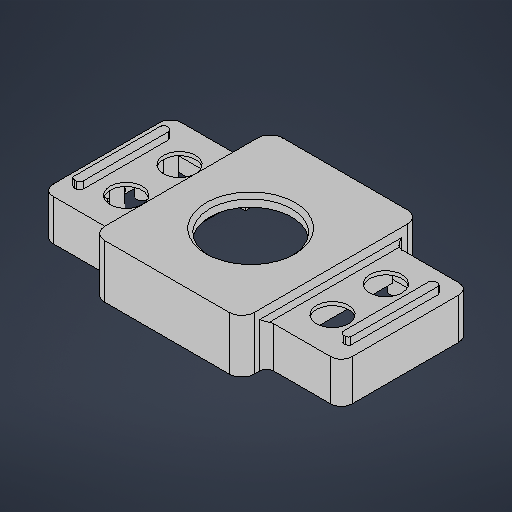
# Autodesk Inventor part: Part1
Saved by Autodesk Inventor 2026 (Build 300175000, 175)
## iProperties
Created: 2025-04-13
Part Number: Part1
Material: Generic
Document SubType Name: Modeling
Designer: ct_vi
Density: 1 g/cm^3
Appearance: Default
Author: ct_vi
Autodesk Inventor part; units mm, degrees
ref_plane "YZ Plane" through (0, 0, 0) normal (1, 0, 0) x (0, 1, 0)
ref_plane "XZ Plane" through (0, 0, 0) normal (0, 1, 0) x (-1, 0, 0)
ref_plane "XY Plane" through (0, 0, 0) normal (0, 0, 1) x (1, 0, 0)
sketch "Sketch1" plane through (0, 0, 0) normal (0, 1, 0) x (-1, 0, 0)
  circle A0 centre (0, 1.5) radius 11.5
  circle A1 centre (0, 1.5) radius 12.5
  line L0 (19.0144, -21.3297) -> (-18.8688, -21.3297) construction
  line L1 (-18.8688, -21.3297) -> (-18.8688, 21.6448) construction
  line L2 (-18.8688, 21.6448) -> (19.0144, 21.6448) construction
  line L3 (19.0144, 21.6448) -> (19.0144, -21.3297) construction
  line L4 (-2.25, -4) -> (-2.25, -8.7)
  line L5 (-2.25, -8.7) -> (2.25, -8.7)
  line L6 (2.25, -8.7) -> (2.25, -4)
  line L7 (2.25, -4) -> (-2.25, -4)
  line L8 (5.9381, 2.2148) -> (9.8353, 4.4648)
  line L9 (9.8353, 4.4648) -> (7.4853, 8.5352)
  line L10 (7.4853, 8.5352) -> (3.5881, 6.2852)
  line L11 (5.9381, 2.2148) -> (3.5881, 6.2852)
  line L12 (-3.5881, 6.2852) -> (-7.4853, 8.5352)
  line L13 (-7.4853, 8.5352) -> (-9.8353, 4.4648)
  line L14 (-9.8353, 4.4648) -> (-5.9381, 2.2148)
  line L15 (-3.5881, 6.2852) -> (-5.9381, 2.2148)
  circle A2 centre (10.199, -17.6855) radius 1.5
  circle A3 centre (-10.301, 18.0645) radius 1.5
  circle A4 centre (10.199, 18.0645) radius 1.5
  circle A5 centre (-10.301, -17.6855) radius 1.5
  line L16 (10.199, -17.6855) -> (-10.301, -17.6855)
  line L17 (-10.301, -17.6855) -> (-10.301, 18.0645)
  line L18 (-10.301, 18.0645) -> (10.199, 18.0645)
  line L19 (10.199, 18.0645) -> (10.199, -17.6855)
  line L20 (18, -22) -> (-18, -22)
  line L21 (-18, -22) -> (-18, 22)
  line L22 (-18, 22) -> (18, 22)
  line L23 (18, 22) -> (18, -22)
  line L24 (18, -22) -> (-18, 22) construction
  line L25 (-18, -22) -> (18, 22) construction
  line L26 (17.5, -25) -> (-17.5, -25)
  line L27 (-21, -21.5) -> (-21, 21.5)
  line L28 (-17.5, 25) -> (17.5, 25)
  line L29 (21, -25) -> (-21, 25) construction
  line L30 (-21, -25) -> (21, 25) construction
  arc A6 (-17.5, 25) -> (-21, 21.5) centre (-17.5, 21.5) ccw
  arc A7 (-21, -21.5) -> (-17.5, -25) centre (-17.5, -21.5) ccw
  line L31 (17.5, -23) -> (-17.5, -23)
  line L32 (-19, -21.5) -> (-19, 21.5)
  line L33 (-17.5, 23) -> (17.5, 23)
  line L34 (19, 21.5) -> (19, -21.5)
  line L35 (19, -23) -> (-19, 23) construction
  line L36 (-19, -23) -> (19, 23) construction
  arc A8 (-17.5, 23) -> (-19, 21.5) centre (-17.5, 21.5) ccw
  arc A9 (-19, -21.5) -> (-17.5, -23) centre (-17.5, -21.5) ccw
  line L37 (9.2678, 19.2405) -> (9.2678, 16.8886)
  line L38 (9.2678, -16.5095) -> (9.2678, -18.8614)
  line L39 (-9.3698, 19.2405) -> (-9.3698, 16.8886)
  line L40 (-9.3698, -16.5095) -> (-9.3698, -18.8614)
  line L41 (17.5, -24) -> (-17.5, -24)
  line L42 (-20, -21.5) -> (-20, 21.5)
  line L43 (-17.5, 24) -> (17.5, 24)
  line L44 (20, -24) -> (-20, 24) construction
  line L45 (-20, -24) -> (20, 24) construction
  arc A10 (-17.5, 24) -> (-20, 21.5) centre (-17.5, 21.5) ccw
  arc A11 (-20, -21.5) -> (-17.5, -24) centre (-17.5, -21.5) ccw
  line L46 (21, -21.5) -> (21, 21.5)
  line L47 (20, 21.5) -> (20, -21.5)
  arc A12 (17.5, -24) -> (20, -21.5) centre (17.5, -21.5) ccw
  arc A13 (17.5, -25) -> (21, -21.5) centre (17.5, -21.5) ccw
  arc A14 (17.5, -23) -> (19, -21.5) centre (17.5, -21.5) ccw
  arc A15 (21, 21.5) -> (17.5, 25) centre (17.5, 21.5) ccw
  arc A16 (20, 21.5) -> (17.5, 24) centre (17.5, 21.5) ccw
  arc A17 (19, 21.5) -> (17.5, 23) centre (17.5, 21.5) ccw
  line L48 (19, -15) -> (19, 15)
  line L49 (19, 16) -> (19, -16)
  line L50 (19, -16) -> (19, 16)
  line L51 (20, -17) -> (20, 17)
  line L52 (21, -18) -> (21, 18)
  line L53 (19, -15) -> (21.5, -15)
  line L54 (21.5, -15) -> (21.5, 16)
  line L55 (21.5, 16) -> (19, 16)
  line L56 (19, 16) -> (19, -15)
  line L57 (-19, -15) -> (-19, 15)
  line L58 (-19, -16) -> (-19, 16)
  line L59 (-21, -18) -> (-21, 19)
  line L60 (-20, -17) -> (-20, 17)
  line L61 (-20, -17) -> (-20, 17)
  line L62 (-19, -16) -> (-19, 16)
  line L63 (-19, 16) -> (-21.5, 16)
  line L64 (-21.5, 16) -> (-21.5, -16)
  line L65 (-21.5, -16) -> (-19, -16)
  line L66 (-19, -16) -> (-19, 16)
  line L67 (14, -15) -> (14, 0)
  line L68 (21, -15) -> (20, -15)
  line L69 (20, -15) -> (20, -16.5095)
  line L70 (21, -16.5095) -> (21, -15)
  line L71 (21, -15) -> (19, -15)
  line L72 (19, -15) -> (19, -16)
  line L73 (19, -16) -> (21, -16)
  line L74 (21, -16) -> (21, -15)
  line L75 (21, -16) -> (19, -16)
  line L76 (19, -16) -> (19, -17)
  line L77 (19, -17) -> (21, -17)
  line L78 (21, -17) -> (21, -16)
  line L79 (21, -17) -> (19, -17)
  line L80 (19, -17) -> (19, -18)
  line L81 (19, -18) -> (21, -18)
  line L82 (21, -18) -> (21, -17)
  line L83 (21, 16) -> (19, 16)
  line L84 (19, 16) -> (19, 18)
  line L85 (19, 18) -> (21, 18)
  line L86 (21, 18) -> (21, 16)
  line L87 (21, 18) -> (19, 18)
  line L88 (19, 18) -> (19, 19)
  line L89 (19, 19) -> (21, 19)
  line L90 (21, 19) -> (21, 18)
  line L91 (21, 18) -> (19, 18)
  line L92 (19, 18) -> (19, 17)
  line L93 (19, 17) -> (21, 17)
  line L94 (21, 17) -> (21, 18)
  line L95 (-19, 16) -> (-21, 16)
  line L96 (-21, 16) -> (-21, 17)
  line L97 (-21, 17) -> (-19, 17)
  line L98 (-19, 17) -> (-19, 16)
  line L99 (-21, 17) -> (-19, 17)
  line L100 (-19, 17) -> (-19, 18)
  line L101 (-19, 18) -> (-21, 18)
  line L102 (-21, 18) -> (-21, 17)
  line L103 (-21, 18) -> (-19, 18)
  line L104 (-19, 18) -> (-19, 19)
  line L105 (-19, 19) -> (-21, 19)
  line L106 (-21, 19) -> (-21, 18)
  line L107 (-19, -16) -> (-21, -16)
  line L108 (-21, -16) -> (-21, -17)
  line L109 (-21, -17) -> (-19, -17)
  line L110 (-19, -17) -> (-19, -16)
  line L111 (-21, -17) -> (-19, -17)
  line L112 (-19, -17) -> (-19, -18)
  line L113 (-19, -18) -> (-21, -18)
  line L114 (-21, -18) -> (-21, -17)
  line L115 (-19, -18) -> (-21, -18)
  line L116 (-21, -18) -> (-21, -19)
  line L117 (-21, -19) -> (-19, -19)
  line L118 (-19, -19) -> (-19, -18)
  point P0 (0, 0)
  point P1 (21, -22)
  point P2 (21, 22)
  point P3 (19, 24)
  point P4 (19, -24)
  point P5 (-21, -16)
  point P6 (-21, 16)
  point P7 (21, 16)
  point P8 (21, -15)
  point P9 (-20, 17)
  point P10 (20, 16)
  point P11 (20, -18)
  dimension "d33" = 4.7
  dimension "d34" = 4.5
  dimension "d36" = 4.5
  dimension "d37" = 4.7
  dimension "d38" = 3
  dimension "d46" = 3
  dimension "d47" = 3
  dimension "d48" = 3
  dimension "d211" = 1.5
  dimension "d212" = 2.5
  dimension "d216" = 3.5
  dimension "d245" = 2.5
  dimension "d246" = 3.5
  dimension "d247" = 1.5
  dimension "d248" = 3.5
  dimension "d249" = 2.5
  dimension "d250" = 1.5
  dimension "d264" = 30
  dimension "d310" = 34
  dimension "d314" = 36
  dimension "d318" = 2.5
  dimension "d366" = 2.5
  dimension "d494" = 2
  dimension "d495" = 1
  dimension "d496" = 2
  dimension "d497" = 1
  dimension "d498" = 2
  dimension "d499" = 1
  dimension "d500" = 2
  dimension "d501" = 1
  dimension "d502" = 1
  dimension "d503" = 1
  dimension "d504" = 1
  dimension "d505" = 1
  dimension "d506" = 1
  dimension "d565" = 50
  constraints: 230 end point, 45 point on line, 39 parallel, 32 point on circle, 27 perpendicular, 24 tangent, 21 horizontal, 18 centre point, 9 midpoint, 1 vertical, 2 other
  measures "d33" distance of L4.start L4.end
  measures "d34" distance of L4.end L5.end
  measures "d36" distance of L8.start L8.end
  measures "d37" distance of L8.end L9.end
  measures "d38" diameter of A2
  measures "d46" diameter of A3
  measures "d47" diameter of A4
  measures "d48" diameter of A5
  measures "d211" radius of A9
  measures "d212" radius of A11
  measures "d216" radius of A7
  measures "d245" radius of A12
  measures "d246" radius of A13
  measures "d247" radius of A14
  measures "d248" radius of A15
  measures "d249" radius of A16
  measures "d250" radius of A17
  measures "d264" distance of L48.start L48.end
  measures "d310" distance of L51.start L51.end
  measures "d314" distance of L52.start L52.end
  measures "d318" distance of L55.end L54.end
  measures "d366" distance of L65.end L64.end
  measures "d494" distance of L73.end L50.start
  measures "d495" distance of L76.end L75.end
  measures "d496" distance of L81.end L80.end
  measures "d497" distance of L80.end L79.end
  measures "d498" distance of L84.end L85.end
  measures "d499" distance of L87.end L88.end
  measures "d500" distance of L96.end L97.end
  measures "d501" distance of L95.end L96.end
  measures "d502" distance of L100.end L99.end
  measures "d503" distance of L104.end L103.end
  measures "d504" distance of L108.end L107.end
  measures "d505" distance of L111.end L112.end
  measures "d506" distance of L116.end L115.end
  measures "d565" distance between parallel lines of L28 L26
extrude "Extrusion40" add sketch "Sketch1" against normal blind 2.5 contours A0 L19 A1 | A0 L17 A1 L19 | L19 A1 L17 A0 | A0 L17 A1
extrude "Extrusion41" add sketch "Sketch1" against normal blind 5 contours L19 L18 L37 A4 | A4 L37 L18 L19 | L19 L16 L38 A2 | A2 L38 L16 L19 | L17 L18 L39 A3 | A3 L39 L18 L17 | L17 L16 L40 A5 | A5 L40 L16 L17
extrude "Spec_Body" add sketch "Sketch1" along normal blind 0.5 and the other way blind 0.75 contours A1 L17 A3 L18 A4 L19 | L19 A2 L16 A5 L17 A1 | L19 L18 L37 A4 | A4 L37 L18 L19 | L19 L16 L38 A2 | A2 L38 L16 L19 | L17 L18 L39 A3 | A3 L39 L18 L17 | A4 L18 L37 | L17 L16 L40 A5 | A5 L40 L16 L17 | L38 L16 A2 | A3 L18 L39 | L39 L18 A3 | A4 L37 L18 | A5 L16 L40 | L40 L16 A5 | A2 L16 L38 | L20 L21 L22 L23 | L26 A7 L27 L117 L42 A11 L41 A12 L47 L81 L46 A13 | L81 L47 L77 L46 | L27 L113 L42 L117 | L77 L47 L73 L46 | L81 L34 L77 L47 | L47 A12 L41 A11 L42 L117 L32 A9 L31 A14 L34 L81 | L27 L109 L42 L113 | L42 L113 L32 L117 | L77 L34 L73 L47 | L34 A14 L31 A9 L32 A8 L33 A17 | L27 L65 L42 L109 | L42 L109 L32 L113 | L73 L47 L53 L46 | L27 L63 L42 L65 | L42 L65 L32 L109 | L53 L47 L55 L46 | L73 L34 L53 L47 | L27 L97 L42 L63 | L42 L63 L32 L65 | L55 L47 L93 L46 | L53 L34 L55 L47 | L27 L101 L42 L97 | L42 L97 L32 L63 | L93 L47 L85 L46 | L55 L34 L93 L47 | L27 L105 L42 L101 | L42 L101 L32 L97 | L85 L47 L89 L46 | L93 L34 L85 L47 | L27 A6 L28 A15 L46 L89 L47 A16 L43 A10 L42 L105 | L42 L105 L32 L101 | L85 L34 L89 L47 | L42 A10 L43 A16 L47 L89 L34 A17 L33 A8 L32 L105
ref_plane "Work Plane3" through (21, 0.5, 18) normal (0, 0, 1) x (1, 0, 0)
ref_plane "Work Plane4" through (21, -3, 18) normal (0, 1, 0) x (1, 0, 0)
sketch "Sketch10" plane through (21, -3, 18) normal (0, 1, 0) x (1, 0, 0)
  line L0 (0, 1) -> (0, 35) projected
  line L1 (0, 35) -> (18, 35)
  line L2 (20, 33) -> (20, 3)
  line L3 (18, 1) -> (0, 1)
  line L4 (0, 1) -> (0, 35)
  arc A0 (20, 33) -> (18, 35) centre (18, 33) ccw
  arc A1 (18, 1) -> (20, 3) centre (18, 3) ccw
  line L5 (0, 0) -> (0, 1) projected
  line L6 (0, 0) -> (18, 0)
  line L7 (21, 3) -> (21, 33)
  line L8 (18, 36) -> (0, 36)
  line L9 (0, 36) -> (0, 0)
  arc A2 (21, 33) -> (18, 36) centre (18, 33) ccw
  arc A3 (18, 0) -> (21, 3) centre (18, 3) ccw
  line L10 (0, 35) -> (0, 34)
  line L11 (0, 34) -> (18, 34)
  line L12 (19, 33) -> (19, 3)
  line L13 (18, 2) -> (0, 2)
  line L14 (0, 2) -> (0, 34)
  line L15 (0, 34) -> (0, 33)
  line L16 (0, 33) -> (18, 33)
  line L17 (18, 33) -> (18, 3)
  line L18 (18, 3) -> (0, 3)
  line L19 (0, 3) -> (0, 33)
  arc A4 (19, 33) -> (18, 34) centre (18, 33) ccw
  arc A5 (18, 2) -> (19, 3) centre (18, 3) ccw
  line L20 (0, 35) -> (0, 34)
  line L21 (0, 34) -> (0, 33)
  line L22 (18, 33) -> (-7, 33)
  line L23 (-7, 33) -> (-7, 18)
  line L24 (-7, 18) -> (18, 18)
  line L25 (18, 18) -> (18, 33)
  line L26 (18, 33) -> (8, 33)
  line L27 (8, 33) -> (8, 25.5)
  line L28 (8, 25.5) -> (18, 25.5)
  line L29 (18, 25.5) -> (18, 33)
  line L30 (18, 18) -> (8, 18)
  line L31 (8, 18) -> (8, 10.5)
  line L32 (8, 10.5) -> (18, 10.5)
  line L33 (18, 10.5) -> (18, 18)
  circle A6 centre (8, 25.5) radius 4.5
  circle A7 centre (8, 10.5) radius 4.5
  line L34 (18, 18) -> (16.8, 18)
  line L35 (17.05, 31) -> (16.55, 31)
  line L36 (15.55, 30) -> (15.55, 6)
  line L37 (16.55, 5) -> (17.05, 5)
  line L38 (18.05, 6) -> (18.05, 30)
  line L39 (18.05, 31) -> (15.55, 5) construction
  line L40 (15.55, 31) -> (18.05, 5) construction
  arc A8 (18.05, 30) -> (17.05, 31) centre (17.05, 30) ccw
  arc A9 (16.55, 31) -> (15.55, 30) centre (16.55, 30) ccw
  arc A10 (17.05, 5) -> (18.05, 6) centre (17.05, 6) ccw
  arc A11 (15.55, 6) -> (16.55, 5) centre (16.55, 6) ccw
  line L41 (18, 33) -> (14.5, 33)
  line L42 (14.5, 33) -> (14.5, 29.5)
  line L43 (14.5, 29.5) -> (18, 29.5)
  line L44 (18, 29.5) -> (18, 33)
  line L45 (18, 18) -> (14.5, 18)
  line L46 (14.5, 18) -> (14.5, 21.5)
  line L47 (14.5, 21.5) -> (18, 21.5)
  line L48 (18, 21.5) -> (18, 18)
  line L49 (18, 18) -> (14.5, 18)
  line L50 (14.5, 18) -> (14.5, 14.5)
  line L51 (14.5, 14.5) -> (18, 14.5)
  line L52 (18, 14.5) -> (18, 18)
  line L53 (18, 3) -> (14.5, 3)
  line L54 (14.5, 3) -> (14.5, 6.5)
  line L55 (14.5, 6.5) -> (18, 6.5)
  line L56 (18, 6.5) -> (18, 3)
  circle A12 centre (14.5, 29.5) radius 1.5
  circle A13 centre (14.5, 21.5) radius 1.5
  circle A14 centre (14.5, 14.5) radius 1.5
  circle A15 centre (14.5, 6.5) radius 1.5
  point P0 (-21, 18)
  point P1 (20, 1)
  point P2 (20, 35)
  point P3 (21, 36)
  point P4 (21, 0)
  point P5 (19, 2)
  point P6 (19, 34)
  point P7 (0, 35)
  point P8 (18, 5.6878)
  point P9 (18, 30.3122)
  dimension "d433" = 20
  dimension "d434" = 34
  dimension "d435" = 2
  dimension "d436" = 21
  dimension "d437" = 36
  dimension "d438" = 3
  dimension "d439" = 1
  dimension "d440" = 19
  dimension "d441" = 32
  dimension "d442" = 1
  dimension "d443" = 1
  dimension "d452" = 25
  dimension "d453" = 15
  dimension "d454" = 10
  dimension "d455" = 7.5
  dimension "d456" = 7.5
  dimension "d457" = 9
  dimension "d458" = 9
  dimension "d529" = 1.2
  dimension "d531" = 26
  dimension "d532" = 2.5
  dimension "d533" = 1
  dimension "d550" = 3.5
  dimension "d551" = 3.5
  dimension "d552" = 3.5
  dimension "d553" = 3.5
  dimension "d554" = 3.5
  dimension "d555" = 3.5
  dimension "d556" = 3.5
  dimension "d557" = 3.5
  dimension "d558" = 3
  dimension "d559" = 3
  dimension "d560" = 3
  dimension "d561" = 3
  constraints: 110 end point, 24 parallel, 24 point on line, 20 point on circle, 20 tangent, 16 centre point, 12 horizontal, 12 perpendicular, 6 coincident, 6 equal radius, 2 collinear, 2 midpoint
  measures "d433" distance of point (20, 1) L3.end
  measures "d434" distance of point (20, 35) point (20, 1)
  measures "d435" radius of A0
  measures "d436" distance of L8.end point (21, 36)
  measures "d437" distance of point (21, 36) point (21, 0)
  measures "d438" radius of A2
  measures "d439" distance of L0.end L10.end
  measures "d440" distance of point (19, 2) L13.end
  measures "d441" distance of point (19, 34) point (19, 2)
  measures "d442" distance of L10.end L15.end
  measures "d443" radius of A4
  measures "d452" distance of L24.end L23.end
  measures "d453" distance of L23.end L22.end
  measures "d454" distance of L28.end L27.end
  measures "d455" distance of L27.end L26.end
  measures "d456" distance of L31.end L30.end
  measures "d457" diameter of A6
  measures "d458" diameter of A7
  measures "d529" distance of L24.end L34.end
  measures "d531" distance of L40.start L39.end
  measures "d532" distance of L39.end L40.end
  measures "d533" radius of A8
  measures "d550" distance of L43.end L42.end
  measures "d551" distance of L42.end L41.end
  measures "d552" distance of L46.end L47.end
  measures "d553" distance of L45.end L46.end
  measures "d554" distance of L51.end L50.end
  measures "d555" distance of L50.end L49.end
  measures "d556" distance of L54.end L55.end
  measures "d557" distance of L53.end L54.end
  measures "d558" diameter of A12
  measures "d559" diameter of A13
  measures "d560" diameter of A14
  measures "d561" diameter of A15
extrude "Extrusion45" add sketch "Sketch10" against normal blind 11.5 contours L3 A1 L2 A0 L1 L9 L8 A2 L7 A3 L6 L5
extrude "Extrusion46" add sketch "Sketch10" against normal blind 6.5 contours L0 L13 A5 L12 A4 L11 L1 A0 L2 A1 L3
extrude "Extrusion47" add sketch "Sketch10" against normal blind 1 contours L0 L18 L17 A10 L38 A8 L16 L11 A4 L12 A5 L13 | L0 L24 L31 A7 L32 L36 A15 L54 L18 | L0 L16 L27 A6 L28 L36 A13 L46 L24 | L54 A15 A11 L37 A10 L17 L18 | L24 L50 A14 L36 L32 A7 L31 | A15 L36 L55 L54 | L54 L55 L36 A11 A15 | L16 L42 A12 L36 L28 A6 L27 | L46 A13 L36 L24 | L24 L36 A14 L50 | A7 L32 L31 | L31 L32 A7 | A10 L37 A11 A15 L55 L17 | L17 A8 L38 A10 | A15 L55 L36 | L36 L32 L17 L55 A15 | A11 L36 L55 A15 | L16 L17 A8 L35 A9 A12 L42 | A6 L28 L27 | L27 L28 A6 | L36 A13 L47 L17 L24 | L24 L17 L51 A14 L36 | A13 L36 L47 L46 | L46 L47 L36 A13 | A14 L36 L51 L50 | L50 L51 L36 A14 | L36 A14 L51 L17 L32 | A12 A9 L36 L43 L42 | L42 L43 L36 A12 | L36 L47 A13 | A14 L51 L36 | A13 L47 L36 | L36 L28 L17 L47 A13 | L36 L51 A14 | L17 L43 A12 A9 L35 A8 | A12 L43 L36 A9 | A12 L43 L17 L28 L36 | L36 L43 A12
extrude "Extrusion49" add sketch "Sketch1" against normal blind 10.3 contours L73 L47 L53 L46 | L27 L63 L42 L65 | L53 L47 L55 L46 | L73 L34 L53 L47 | L42 L63 L32 L65 | L53 L34 L55 L47
extrude "Extrusion50" cut sketch "Sketch10" along normal through all both and the other way through all contours A7 L32 L31 | L31 L32 A7 | A6 L28 L27 | L27 L28 A6
sketch "Sketch11" plane through (21, -3, 18) normal (0, 1, 0) x (1, 0, 0)
  line L0 (-21, 18) -> (-42, 18)
  line L1 (-42, 39.5) -> (-42, -3.5) projected
  line L2 (-42, 18) -> (-42, 36)
  line L3 (-42, 36) -> (-60, 36)
  line L4 (-63, 33) -> (-63, 3)
  line L5 (-60, 0) -> (-42, 0)
  line L6 (-42, 0) -> (-42, 36)
  line L7 (-42, 36) -> (-42, 35)
  line L8 (-42, 35) -> (-60, 35)
  line L9 (-62, 33) -> (-62, 3)
  line L10 (-60, 1) -> (-42, 1)
  line L11 (-42, 1) -> (-42, 35)
  line L12 (-42, 35) -> (-42, 34)
  line L13 (-42, 34) -> (-60, 34)
  line L14 (-61, 33) -> (-61, 3)
  line L15 (-60, 2) -> (-42, 2)
  line L16 (-42, 2) -> (-42, 34)
  line L17 (-42, 34) -> (-42, 33)
  line L18 (-42, 33) -> (-60, 33)
  line L19 (-60, 33) -> (-60, 3)
  line L20 (-60, 3) -> (-42, 3)
  line L21 (-42, 3) -> (-42, 33)
  arc A0 (-63, 3) -> (-60, 0) centre (-60, 3) ccw
  arc A1 (-60, 36) -> (-63, 33) centre (-60, 33) ccw
  arc A2 (-60, 35) -> (-62, 33) centre (-60, 33) ccw
  arc A3 (-62, 3) -> (-60, 1) centre (-60, 3) ccw
  arc A4 (-61, 3) -> (-60, 2) centre (-60, 3) ccw
  arc A5 (-60, 34) -> (-61, 33) centre (-60, 33) ccw
  line L22 (-60, 3) -> (-50, 3)
  line L23 (-50, 3) -> (-50, 10.5)
  line L24 (-50, 10.5) -> (-60, 10.5)
  line L25 (-60, 10.5) -> (-60, 3)
  line L26 (-60, 33) -> (-50, 33)
  line L27 (-50, 33) -> (-50, 25.5)
  line L28 (-50, 25.5) -> (-60, 25.5)
  line L29 (-60, 25.5) -> (-60, 33)
  circle A6 centre (-50, 10.5) radius 4.5
  circle A7 centre (-50, 25.5) radius 4.5
  line L30 (-60, 3) -> (-60, 18)
  line L31 (-60, 18) -> (-58.8, 18)
  line L32 (-59.05, 31) -> (-58.55, 31)
  line L33 (-57.55, 30) -> (-57.55, 6)
  line L34 (-58.55, 5) -> (-59.05, 5)
  line L35 (-60.05, 6) -> (-60.05, 30)
  line L36 (-60.05, 31) -> (-57.55, 5) construction
  line L37 (-57.55, 31) -> (-60.05, 5) construction
  arc A8 (-58.55, 5) -> (-57.55, 6) centre (-58.55, 6) ccw
  arc A9 (-60.05, 6) -> (-59.05, 5) centre (-59.05, 6) ccw
  arc A10 (-57.55, 30) -> (-58.55, 31) centre (-58.55, 30) ccw
  arc A11 (-59.05, 31) -> (-60.05, 30) centre (-59.05, 30) ccw
  line L38 (-60, 3) -> (-56.5, 3)
  line L39 (-56.5, 3) -> (-56.5, 6.5)
  line L40 (-56.5, 6.5) -> (-60, 6.5)
  line L41 (-60, 6.5) -> (-60, 3)
  line L42 (-60, 33) -> (-56.5, 33)
  line L43 (-56.5, 33) -> (-56.5, 29.5)
  line L44 (-56.5, 29.5) -> (-60, 29.5)
  line L45 (-60, 29.5) -> (-60, 33)
  circle A12 centre (-56.5, 29.5) radius 1.5
  circle A13 centre (-56.5, 6.5) radius 1.5
  line L46 (-60, 18) -> (-56.5, 18)
  line L47 (-56.5, 18) -> (-56.5, 21.5)
  line L48 (-56.5, 21.5) -> (-60, 21.5)
  line L49 (-60, 21.5) -> (-60, 18)
  circle A14 centre (-56.5, 21.5) radius 1.5
  line L50 (-59.9732, 18) -> (-56.4732, 18)
  line L51 (-56.4732, 18) -> (-56.4732, 14.5)
  line L52 (-56.4732, 14.5) -> (-59.9732, 14.5)
  line L53 (-59.9732, 14.5) -> (-59.9732, 18)
  circle A15 centre (-56.4732, 14.5) radius 1.5
  point P0 (-63, 0)
  point P1 (-63, 36)
  point P2 (-62, 1)
  point P3 (-62, 35)
  point P4 (-61, 2)
  point P5 (-61, 34)
  point P6 (-42, 0)
  point P7 (-42, 1)
  point P8 (-42, 2)
  point P9 (-58.8, 7.4624)
  point P10 (-58.8, 28.5376)
  point P11 (-60, 30.3122)
  point P12 (-60, 5.6878)
  dimension "d465" = 18
  dimension "d466" = 21
  dimension "d467" = 36
  dimension "d468" = 1
  dimension "d469" = 20
  dimension "d470" = 34
  dimension "d471" = 1
  dimension "d472" = 19
  dimension "d473" = 32
  dimension "d474" = 1
  dimension "d475" = 18
  dimension "d476" = 30
  dimension "d477" = 3
  dimension "d478" = 2
  dimension "d479" = 1
  dimension "d486" = 10
  dimension "d487" = 7.5
  dimension "d488" = 10
  dimension "d489" = 7.5
  dimension "d490" = 9
  dimension "d491" = 9
  dimension "d524" = 1.2
  dimension "d525" = 2.5
  dimension "d526" = 1
  dimension "d530" = 26
  dimension "d536" = 3.5
  dimension "d537" = 3.5
  dimension "d538" = 3.5
  dimension "d539" = 3.5
  dimension "d540" = 3
  dimension "d541" = 3
  dimension "d544" = 3.5
  dimension "d545" = 3.5
  dimension "d546" = 3
  dimension "d547" = 3.5
  dimension "d548" = 3.5
  dimension "d549" = 3
  constraints: 106 end point, 25 point on line, 22 parallel, 20 point on circle, 20 tangent, 16 centre point, 12 perpendicular, 11 horizontal, 6 coincident, 6 equal radius, 4 midpoint
  measures "d465" distance of L0.end L2.end
  measures "d466" distance of L5.end point (-63, 0)
  measures "d467" distance of point (-63, 0) point (-63, 36)
  measures "d468" distance of L2.end L7.end
  measures "d469" distance of L10.end point (-62, 1)
  measures "d470" distance of point (-62, 1) point (-62, 35)
  measures "d471" distance of L7.end L12.end
  measures "d472" distance of L15.end point (-61, 2)
  measures "d473" distance of point (-61, 2) point (-61, 34)
  measures "d474" distance of L12.end L17.end
  measures "d475" distance of L20.end L19.end
  measures "d476" distance of L19.end L18.end
  measures "d477" radius of A0
  measures "d478" radius of A2
  measures "d479" radius of A4
  measures "d486" distance of L24.end L23.end
  measures "d487" distance of L23.end L22.end
  measures "d488" distance of L27.end L28.end
  measures "d489" distance of L26.end L27.end
  measures "d490" diameter of A6
  measures "d491" diameter of A7
  measures "d524" distance of L30.end L31.end
  measures "d525" distance of L36.end L37.end
  measures "d526" radius of A8
  measures "d530" distance between parallel lines of L32 L34
  measures "d536" distance of L40.end L39.end
  measures "d537" distance of L39.end L38.end
  measures "d538" distance of L43.end L44.end
  measures "d539" distance of L42.end L43.end
  measures "d540" diameter of A12
  measures "d541" diameter of A13
  measures "d544" distance of L48.end L47.end
  measures "d545" distance of L47.end L46.end
  measures "d546" diameter of A14
  measures "d547" distance of L51.end L52.end
  measures "d548" distance of L50.end L51.end
  measures "d549" diameter of A15
extrude "Extrusion51" add sketch "Sketch11" against normal blind 11.5 contours L1 L8 A2 L9 A3 L10 L5 A0 L4 A1 L3
extrude "Extrusion52" add sketch "Sketch11" against normal blind 6.5 contours L1 L13 A5 L14 A4 L15 L10 A3 L9 A2 L8
extrude "Extrusion53" add sketch "Sketch11" against normal blind 1 contours L1 L18 L19 A11 L35 A9 L20 L15 A4 L14 A5 L13 | L1 L20 L23 A6 L24 L33 A15 L51 L50 L47 A14 L28 A7 L27 L18 | L27 A7 L28 L33 A12 L43 L18 | L43 A12 A10 L32 A11 L19 L18 | A7 L28 L27 | L27 L28 A7 | L20 L39 A13 L33 L24 A6 L23 | A12 L33 L44 L43 | L43 L44 L33 A10 A12 | L20 L19 A9 L34 A8 A13 L39 | A6 L24 L23 | L23 L24 A6 | A11 L32 A10 A12 L44 L19 | L19 A9 L35 A11 | A10 L33 L44 A12 | L33 A14 L48 L19 L28 | L28 L19 L44 A12 L33 | A13 A8 L33 L40 L39 | L39 L40 L33 A13 | L33 A12 L44 | A14 L47 L48 L33 | L33 L48 A14 | L19 L40 A13 A8 L34 A9 | A13 L40 L33 A8 | L33 A13 L40 L19 L24 | L24 L19 L31 L53 L52 A15 L33 | L48 A14 L33 L46 L31 L19 | L48 L47 A14 L33 | L33 A14 L48 | L40 A13 L33 | A15 L52 L33 | L33 L52 L51 A15 | A14 L47 L46 L33 | L52 A15 L33 | L33 A15 L51 L52 | L52 L53 L31 L46 L33 A15 | L46 L50 L51 A15 L33
extrude "Extrusion54" cut sketch "Sketch11" along normal through all both and the other way through all contours A7 L28 L27 | L27 L28 A7 | A6 L24 L23 | L23 L24 A6
extrude "Extrusion55" add sketch "Sketch1" against normal blind 9.5 contours L77 L47 L73 L46 | L81 L34 L77 L47 | L47 A12 L41 A11 L42 L117 L32 A9 L31 A14 L34 L81 | L42 L113 L32 L117 | L77 L34 L73 L47 | L27 L65 L42 L109 | L42 L109 L32 L113 | L42 L65 L32 L109 | L27 L97 L42 L63 | L55 L47 L93 L46 | L42 L97 L32 L63 | L55 L34 L93 L47 | L42 L101 L32 L97 | L93 L34 L85 L47 | L42 L105 L32 L101 | L85 L34 L89 L47 | L42 A10 L43 A16 L47 L89 L34 A17 L33 A8 L32 L105
extrude "Extrusion56" add sketch "Sketch1" against normal blind 14.5 contours L26 A7 L27 L117 L42 A11 L41 A12 L47 L81 L46 A13 | L81 L47 L77 L46 | L27 L113 L42 L117 | L27 L109 L42 L113 | L27 L101 L42 L97 | L93 L47 L85 L46 | L27 L105 L42 L101 | L85 L47 L89 L46 | L27 A6 L28 A15 L46 L89 L47 A16 L43 A10 L42 L105
sketch "Sketch12" plane through (-21, 0.5, -21.5) normal (-1, 0, 0) x (0, 0, 1)
  line L0 (37.5, -4.5) -> (37.5, -10.8) projected
  line L1 (37.5, -10.8) -> (5.5, -10.8) projected
  line L2 (37.5, -4.5) -> (5.5, -4.5)
  line L3 (5.5, -4.5) -> (5.5, -10.8)
  line L4 (5.5, -10.8) -> (37.5, -10.8)
  line L5 (37.5, -10.8) -> (37.5, -4.5)
  point P0 (21.5, -0.5)
  point P1 (37.5, -10)
  point P2 (37.5, -10.5)
  dimension "d511" = 6.3
  constraints: 8 end point, 2 parallel, 1 horizontal, 1 perpendicular
  measures "d511" distance of L1.end L2.end
extrude "Extrusion57" add sketch "Sketch12" along normal blind 1
sketch "Sketch13" plane through (21, -10.3, 16) normal (1, 0, 0) x (0, 0, -1)
  line L0 (32, 6.3) -> (32, 0.8) projected
  line L1 (32, 0) -> (0, 0) projected
  line L2 (32, 6.3) -> (0, 6.3)
  line L3 (0, 6.3) -> (0, 0)
  line L4 (0, 0) -> (32, 0)
  line L5 (32, 0) -> (32, 6.3)
  point P0 (16, 10.3)
  constraints: 8 end point, 2 parallel, 1 horizontal, 1 perpendicular
extrude "Extrusion58" add sketch "Sketch13" along normal blind 1.5
fillet "Fillet13" radius 2 4 edges at (21, -8.75, 18) (-21, -8.75, 18) (-21, -8.75, -18) (21, -8.75, -18)
fillet "Fillet14" radius 1 4 edges at (21, -3, -19) (21, -3, 19) (-21, -3, -19) (-21, -3, 19)
chamfer "Chamfer4" distance 0.5 angle 45 1 edges at (12.5, 0, 1.5)
chamfer "Chamfer5" distance 0.5 angle 45 1 edges at (11.5, 0, 1.5)
extrude "Extrusion59" add sketch "Sketch11" along normal blind 2 contours A11 L32 A10 A12 L44 L19 | A10 L33 L44 A12 | L33 A14 L48 L19 L28 | L28 L19 L44 A12 L33 | L33 A12 L44 | L33 L48 A14 | L19 L40 A13 A8 L34 A9 | A13 L40 L33 A8 | L33 A13 L40 L19 L24 | L24 L19 L31 L53 L52 A15 L33 | L48 A14 L33 L46 L31 L19 | L33 A14 L48 | L40 A13 L33 | A15 L52 L33 | L52 A15 L33 | L52 L53 L31 L46 L33 A15
extrude "Extrusion60" add sketch "Sketch10" along normal blind 2 contours A10 L37 A11 A15 L55 L17 | A15 L55 L36 | L36 L32 L17 L55 A15 | A11 L36 L55 A15 | L36 A13 L47 L17 L24 | L24 L17 L51 A14 L36 | L36 A14 L51 L17 L32 | L36 L47 A13 | A14 L51 L36 | A13 L47 L36 | L36 L28 L17 L47 A13 | L36 L51 A14 | L17 L43 A12 A9 L35 A8 | A12 L43 L36 A9 | A12 L43 L17 L28 L36 | L36 L43 A12
extrude "Extrusion61" add sketch "Sketch11" against normal blind 9 contours A12 L33 L44 L43 | L43 L44 L33 A10 A12 | A10 L33 L44 A12 | A13 A8 L33 L40 L39 | L39 L40 L33 A13 | L33 A12 L44 | A14 L47 L48 L33 | L33 L48 A14 | A13 L40 L33 A8 | L48 L47 A14 L33 | L33 A14 L48 | L40 A13 L33 | A15 L52 L33 | L33 L52 L51 A15 | L52 A15 L33 | L33 A15 L51 L52
extrude "Extrusion62" add sketch "Sketch10" against normal blind 9 contours A15 L36 L55 L54 | L54 L55 L36 A11 A15 | A15 L55 L36 | A11 L36 L55 A15 | A13 L36 L47 L46 | L46 L47 L36 A13 | A14 L36 L51 L50 | L50 L51 L36 A14 | A12 A9 L36 L43 L42 | L42 L43 L36 A12 | L36 L47 A13 | A14 L51 L36 | A13 L47 L36 | L36 L51 A14 | A12 L43 L36 A9 | L36 L43 A12
sketch "Sketch17" plane through (17.5, -9.5, 24) normal (0, 0, -1) x (-1, 0, 0)
  line L0 (0, 0) -> (0, -5) projected
  line L1 (0, -5) -> (17.5, -5)
  line L2 (35, -5) -> (0, -5) projected
  line L3 (0, -5) -> (17.5, -5) construction
  line L4 (17.5, -5) -> (17.5, -3)
  line L5 (17.5, -5) -> (19.5, -5) construction
  line L6 (20, -2) -> (15, -2)
  line L7 (15, -2) -> (15, -4)
  line L8 (15, -4) -> (20, -4)
  line L9 (20, -4) -> (20, -2)
  line L10 (20, -2) -> (15, -4) construction
  line L11 (15, -2) -> (20, -4) construction
  point P0 (17.5, 9.5)
  dimension "d575" = 17.5
  dimension "d576" = 0
  dimension "d577" = 2
  dimension "d578" = 90
  dimension "d579" = 5
  dimension "d580" = 2
  constraints: 20 end point, 3 horizontal, 2 equal length, 2 midpoint, 2 parallel, 1 collinear, 1 perpendicular, 1 vertical
  measures "d575" distance of L0.end L1.end
  measures "d576" distance between parallel lines of L1 L3
  measures "d577" distance of L3.end L4.end
  measures "d578" angle of L5 L4
  measures "d579" distance of L8.end L7.end
  measures "d580" distance of L7.end L6.end
extrude "Extrusion63" add sketch "Sketch17" along normal blind 1.75
chamfer "Chamfer6" distance 1.5 angle 40 1 edges at (0, -13.5, 22.25) measured on face at (0.8333, -13.5, 23.4167)
sketch "Sketch18" plane through (-17.5, -9.5, -24) normal (0, 0, 1) x (1, 0, 0)
  line L0 (35, -5) -> (0, -5) projected
  line L1 (0, -5) -> (17.5, -5)
  line L2 (0, -5) -> (17.5, -5) construction
  line L3 (17.5, -5) -> (17.5, -3)
  line L4 (20, -4) -> (15, -4)
  line L5 (15, -4) -> (15, -2)
  line L6 (15, -2) -> (20, -2)
  line L7 (20, -2) -> (20, -4)
  line L8 (20, -4) -> (15, -2) construction
  line L9 (15, -4) -> (20, -2) construction
  point P0 (17.5, 9.5)
  dimension "d586" = 17.5
  dimension "d587" = 0
  dimension "d588" = 2
  dimension "d589" = 90
  dimension "d590" = 5
  dimension "d591" = 2
  constraints: 18 end point, 2 collinear, 2 horizontal, 2 midpoint, 2 parallel, 2 perpendicular
  measures "d586" distance of L0.end L1.end
  measures "d587" distance between parallel lines of L1 L2
  measures "d588" distance of L1.end L3.end
  measures "d589" angle of L3 L1
  measures "d590" distance of L5.end L6.end
  measures "d591" distance of L4.end L5.end
extrude "Extrusion64" add sketch "Sketch18" along normal blind 1.75
chamfer "Chamfer7" distance 1.5 angle 40 1 edges at (0, -13.5, -22.25) measured on face at (-0.8333, -13.5, -23.4167)
sketch "Sketch19" plane through (41, -14.5, -15) normal (-1, 0, 0) x (0, 0, 1)
  line L0 (0, 5) -> (0, 0) projected
  line L1 (0, 0) -> (15, 0)
  line L2 (0, 0) -> (15, 0) construction
  line L3 (15, 0) -> (15, 2)
  line L4 (17.5, 3) -> (12.5, 3)
  line L5 (12.5, 3) -> (12.5, 1)
  line L6 (12.5, 1) -> (17.5, 1)
  line L7 (17.5, 1) -> (17.5, 3)
  line L8 (17.5, 3) -> (12.5, 1) construction
  line L9 (12.5, 3) -> (17.5, 1) construction
  point P0 (15, 14.5)
  dimension "d597" = 15
  dimension "d598" = 0
  dimension "d599" = 2
  dimension "d600" = 90
  dimension "d601" = 5
  dimension "d602" = 2
  constraints: 18 end point, 3 horizontal, 2 midpoint, 2 parallel, 2 perpendicular, 1 collinear
  measures "d597" distance of L0.end L1.end
  measures "d598" distance between parallel lines of L1 L2
  measures "d599" distance of L1.end L3.end
  measures "d600" angle of L3 L1
  measures "d601" distance of L6.end L5.end
  measures "d602" distance of L5.end L4.end
extrude "Extrusion65" add sketch "Sketch19" along normal blind 1.75
chamfer "Chamfer8" distance 1.5 angle 40 1 edges at (39.25, -13.5, 0) measured on face at (39.8333, -13.5, -0.8333)
sketch "Sketch20" plane through (-41, -14.5, 15) normal (1, 0, 0) x (0, 0, -1)
  line L0 (0, 5) -> (0, 0) projected
  line L1 (0, 0) -> (15, 0)
  line L2 (0, 0) -> (15, 0) construction
  line L3 (15, 0) -> (15, 2)
  line L4 (30, 0) -> (0, 0) projected
  line L5 (17.5, 1) -> (12.5, 1)
  line L6 (12.5, 1) -> (12.5, 3)
  line L7 (12.5, 3) -> (17.5, 3)
  line L8 (17.5, 3) -> (17.5, 1)
  line L9 (17.5, 1) -> (12.5, 3) construction
  line L10 (12.5, 1) -> (17.5, 3) construction
  point P0 (15, 14.5)
  dimension "d608" = 15
  dimension "d609" = 0
  dimension "d610" = 2
  dimension "d611" = 90
  dimension "d612" = 5
  dimension "d613" = 2
  constraints: 18 end point, 3 horizontal, 2 midpoint, 2 parallel, 2 perpendicular, 1 collinear
  measures "d608" distance of L0.end L1.end
  measures "d609" distance between parallel lines of L1 L2
  measures "d610" distance of L1.end L3.end
  measures "d611" angle of L3 L1
  measures "d612" distance of L6.end L7.end
  measures "d613" distance of L5.end L6.end
extrude "Extrusion66" add sketch "Sketch20" along normal blind 1.75
chamfer "Chamfer9" distance 1.5 angle 40 1 edges at (-39.25, -13.5, 0) measured on face at (-39.8333, -13.5, 0.8333)
sketch "Sketch22" plane through (-22, 0.5, -21.5) normal (-1, 0, 0) x (0, 0, 1)
  line L0 (5.5, -4.5) -> (37.5, -4.5) projected
  line L1 (37.5, -10.8) -> (37.5, -10) projected
  line L2 (5.5, -4.5) -> (37.5, -4.5)
  line L3 (37.5, -4.5) -> (37.5, -10.8)
  line L4 (37.5, -10.8) -> (5.5, -10.8)
  line L5 (5.5, -10.8) -> (5.5, -4.5)
  point P0 (21.5, -0.5)
  constraints: 8 end point, 2 parallel, 1 horizontal, 1 perpendicular
extrude "Extrusion67" add sketch "Sketch22" along normal blind 0.5
body "Solid2"
